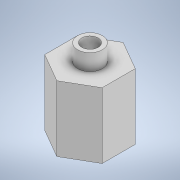
# Autodesk Inventor part: pipeJoint
Saved by Autodesk Inventor 2021 (Build 250183000, 183)
## iProperties
Created: 2021-01-06
Part Number: pipeJoint
Material: Generic
Document SubType Name: Modeling
Designer: awitc
Density: 1 g/cm^3
Appearance: Default
Author: awitc
Autodesk Inventor part; units mm, degrees
ref_plane "YZ Plane" through (0, 0, 0) normal (1, 0, 0) x (0, 1, 0)
ref_plane "XZ Plane" through (0, 0, 0) normal (0, 1, 0) x (-1, 0, 0)
ref_plane "XY Plane" through (0, 0, 0) normal (0, 0, 1) x (1, 0, 0)
sketch "Sketch1" plane through (0, 0, 0) normal (0, 1, 0) x (-1, 0, 0)
  line L0 (3.5, -2.0207) -> (0, -4.0415)
  line L1 (0, -4.0415) -> (-3.5, -2.0207)
  line L2 (-3.5, -2.0207) -> (-3.5, 2.0207)
  line L3 (-3.5, 2.0207) -> (0, 4.0415)
  line L4 (0, 4.0415) -> (3.5, 2.0207)
  line L5 (3.5, 2.0207) -> (3.5, -2.0207)
  circle A0 centre (0, 0) radius 2.5
  point P0 (3.5, 0)
  dimension "d1" = 5
  constraints: 12 end point, 1 centre point, 1 coincident, 1 midpoint, 13 other
  measures "d1" diameter of A0
extrude "Extrusion1" add sketch "Sketch1" along normal blind 5
thread "Thread1" size "M5x0.8" class "6H" standard "ANSI Metric M Profile" full length
sketch "Sketch2" plane through (0, 5, 0) normal (0, 1, 0) x (1, 0, 0)
  circle A0 centre (0, 0) radius 2.5 projected
  line L0 (-3.5, 2.0207) -> (-3.5, -2.0207) projected
  line L1 (-3.5, 2.0207) -> (0, 4.0415)
  line L2 (0, 4.0415) -> (3.5, 2.0207)
  line L3 (3.5, 2.0207) -> (3.5, -2.0207)
  line L4 (3.5, -2.0207) -> (0, -4.0415)
  line L5 (0, -4.0415) -> (-3.5, -2.0207)
  line L6 (-3.5, -2.0207) -> (-3.5, 2.0207)
  point P0 (-3.5, 0)
  constraints: 12 end point, 2 midpoint, 1 coincident, 13 other
extrude "Extrusion2" add sketch "Sketch2" along normal blind 3 contours A0 | L1 L2 L3 L4 L5 L0
sketch "Sketch3" plane through (0, 8, 0) normal (0, 1, 0) x (1, 0, 0)
  circle A0 centre (0, 0) radius 1
  circle A1 centre (0, 0) radius 1.5
  dimension "d8" = 2
  dimension "d9" = 3
  constraints: 2 centre point, 2 coincident
  measures "d8" diameter of A0
  measures "d9" diameter of A1
extrude "Extrusion3" add sketch "Sketch3" along normal blind 2
extrude "Extrusion4" cut sketch "Sketch3" against normal up to next contours A0 | A1
body "Solid1"
